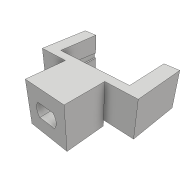
# Autodesk Inventor part: sensor holder
Saved by Autodesk Inventor 2018.3 (Build 223284000, 284)
## iProperties
Created: 2020-03-05
Part Number: sensor holder
Material: Generic
Document SubType Name: Modeling
Designer: Erik
Density: 1 g/cm^3
Appearance: Default
Author: Erik
Autodesk Inventor part; units mm, degrees
ref_plane "YZ Plane" through (0, 0, 0) normal (1, 0, 0) x (0, 1, 0)
ref_plane "XZ Plane" through (0, 0, 0) normal (0, 1, 0) x (-1, 0, 0)
ref_plane "XY Plane" through (0, 0, 0) normal (0, 0, 1) x (1, 0, 0)
sketch "Sketch1" plane through (0, 0, 0) normal (0, 1, 0) x (-1, 0, 0)
  line L0 (5, 5) -> (-5, 5)
  line L1 (-5, 5) -> (-5, -5)
  line L2 (-5, -5) -> (5, -5)
  line L3 (5, -5) -> (5, 5)
  line L4 (5, 5) -> (-5, -5) construction
  line L5 (-5, 5) -> (5, -5) construction
  point P0 (0, 0)
  dimension "d1" = 10
  dimension "d2" = 10
  constraints: 12 end point, 2 midpoint, 2 parallel, 1 horizontal, 1 perpendicular
  measures "d1" distance of L2.end L1.end
  measures "d2" distance of L1.end L0.end
extrude "Extrusion1" add sketch "Sketch1" along normal blind 9
sketch "Sketch2" plane through (0, 9, 0) normal (0, 1, 0) x (1, 0, 0)
  line L0 (-12, 3.5) -> (12, 3.5)
  line L1 (12, 3.5) -> (12, -3.5)
  line L2 (12, -3.5) -> (-12, -3.5)
  line L3 (-12, -3.5) -> (-12, 3.5)
  line L4 (-12, 3.5) -> (12, -3.5) construction
  line L5 (12, 3.5) -> (-12, -3.5) construction
  point P0 (0, 0)
  dimension "d5" = 24
  dimension "d6" = 7
  constraints: 12 end point, 2 midpoint, 2 parallel, 1 horizontal, 1 perpendicular
  measures "d5" distance of L1.end L2.end
  measures "d6" distance of L0.end L1.end
extrude "Extrusion2" add sketch "Sketch2" along normal blind 12
sketch "Sketch3" plane through (0, 21, 0) normal (0, 1, 0) x (1, 0, 0)
  line L0 (-9, -0.65) -> (9, -0.65)
  line L1 (9, -0.65) -> (9, 0.65)
  line L2 (9, 0.65) -> (-9, 0.65)
  line L3 (-9, 0.65) -> (-9, -0.65)
  line L4 (-9, -0.65) -> (9, 0.65) construction
  line L5 (9, -0.65) -> (-9, 0.65) construction
  point P0 (0, 0)
  dimension "d9" = 18
  dimension "d10" = 1.3
  constraints: 12 end point, 2 midpoint, 2 parallel, 1 horizontal, 1 perpendicular
  measures "d9" distance of L2.end L1.end
  measures "d10" distance of L1.end L0.end
extrude "Extrusion3" cut sketch "Sketch3" against normal blind 10 draft 3
sketch "Sketch4" plane through (0, 21, 0) normal (0, 1, 0) x (1, 0, 0)
  line L0 (8.7, -5.0478) -> (-8.7, -5.0478)
  line L1 (-8.7, -5.0478) -> (-8.7, 5.0478)
  line L2 (-8.7, 5.0478) -> (8.7, 5.0478)
  line L3 (8.7, 5.0478) -> (8.7, -5.0478)
  line L4 (8.7, -5.0478) -> (-8.7, 5.0478) construction
  line L5 (-8.7, -5.0478) -> (8.7, 5.0478) construction
  line L6 (-9, -0.65) -> (-9, 0.65) projected
  point P0 (0, 0)
  dimension "d13" = 0.3
  constraints: 12 end point, 2 midpoint, 2 parallel, 1 horizontal, 1 perpendicular
  measures "d13" distance between parallel lines of L1 L6
extrude "Extrusion4" cut sketch "Sketch4" against normal blind 10
sketch "Sketch5" plane through (0, 0, 0) normal (0, -1, 0) x (1, 0, 0)
  circle A0 centre (0, 0) radius 2.65
  dimension "d16" = 5.3
  constraints: 1 centre point, 1 coincident
  measures "d16" diameter of A0
extrude "Extrusion5" cut sketch "Sketch5" against normal blind 7.5 draft -1
sketch "Sketch6" plane through (0, 0, 0) normal (0, -1, 0) x (1, 0, 0)
  line L0 (3.5, 1.7) -> (-3.5, 1.7)
  line L1 (-3.5, 1.7) -> (-3.5, -1.7)
  line L2 (-3.5, -1.7) -> (3.5, -1.7)
  line L3 (3.5, -1.7) -> (3.5, 1.7)
  line L4 (3.5, 1.7) -> (-3.5, -1.7) construction
  line L5 (-3.5, 1.7) -> (3.5, -1.7) construction
  line L6 (3.9892, 3.699) -> (-3.9892, 3.699)
  line L7 (-3.9892, 3.699) -> (-3.9892, -3.699)
  line L8 (-3.9892, -3.699) -> (3.9892, -3.699)
  line L9 (3.9892, -3.699) -> (3.9892, 3.699)
  line L10 (3.9892, 3.699) -> (-3.9892, -3.699) construction
  line L11 (-3.9892, 3.699) -> (3.9892, -3.699) construction
  point P0 (0, 0)
  dimension "d19" = 3.4
  dimension "d20" = 7
  constraints: 24 end point, 4 midpoint, 4 parallel, 2 horizontal, 2 perpendicular
  measures "d19" distance of L1.end L0.end
  measures "d20" distance between parallel lines of L1 L3
extrude "Extrusion6" add sketch "Sketch6" against normal blind 7.5 draft 1.5
sketch "Sketch7" plane through (-12, 9, 3.5) normal (0, 0, 1) x (1, 0, 0)
  line L0 (20.7, 12) -> (20.7, 2) projected
  line L1 (20.7, 2) -> (3.3, 2) projected
  line L2 (3.3, 2) -> (3.3, 12) projected
  line L3 (0, 12) -> (3.3, 12) projected
  line L4 (0, 0) -> (0, 12) projected
  line L5 (7, 0) -> (0, 0) projected
  line L6 (17, 0) -> (7, 0) projected
  line L7 (24, 0) -> (17, 0) projected
  line L8 (24, 0) -> (24, 12) projected
  line L9 (20.7, 12) -> (24, 12) projected
  point P0 (12, -9)
extrude "Extrusion7" add sketch "Sketch7" along normal up to surface (1.5 mm away)
body "Solid1"
